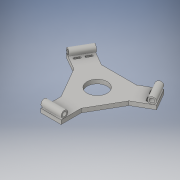
# Autodesk Inventor part: end effector
Saved by Autodesk Inventor 2016 (Build 200138000, 138)
## iProperties
Created: 2016-04-21
Part Number: end effector
Material: Generic
Document SubType Name: Modeling
Designer: Sam
Density: 1 g/cm^3
Appearance: Default
Author: Sam
Autodesk Inventor part; units mm, degrees
ref_plane "YZ Plane" through (0, 0, 0) normal (1, 0, 0) x (0, 1, 0)
ref_plane "XZ Plane" through (0, 0, 0) normal (0, 1, 0) x (-1, 0, 0)
ref_plane "XY Plane" through (0, 0, 0) normal (0, 0, 1) x (1, 0, 0)
sketch "Sketch1" plane through (0, 0, 0) normal (0, 1, 0) x (-1, 0, 0)
  line L0 (-7.5, 19.3301) -> (-7.5, 34.3301)
  line L1 (-7.5, 34.3301) -> (7.5, 34.3301)
  line L2 (7.5, 34.3301) -> (7.5, 19.3301)
  line L3 (20.4904, -3.1699) -> (33.4808, -10.6699)
  line L4 (33.4808, -10.6699) -> (25.9808, -23.6603)
  line L5 (25.9808, -23.6603) -> (12.9904, -16.1603)
  line L6 (-12.9904, -16.1603) -> (-25.9808, -23.6603)
  line L7 (-25.9808, -23.6603) -> (-33.4808, -10.6699)
  line L8 (-33.4808, -10.6699) -> (-20.4904, -3.1699)
  line L9 (7.5, 19.3301) -> (20.4904, -3.1699)
  line L10 (12.9904, -16.1603) -> (-12.9904, -16.1603)
  line L11 (-20.4904, -3.1699) -> (-7.5, 19.3301)
  point P0 (0, 0)
  point P1 (0, 0)
  constraints: 24 end point, 6 perpendicular, 1 coincident, 1 vertical, 1 other
extrude "Extrusion1" add sketch "Sketch1" along normal blind 3
sketch "Sketch2" plane through (0, 3, 0) normal (0, 1, 0) x (1, 0, 0)
  circle A0 centre (0, 0) radius 7.5
  line L0 (33.4808, 10.6699) -> (25.9808, 23.6603) projected
  line L1 (29.7308, 17.1651) -> (35.4808, 17.1651) construction
  line L2 (20.4904, 3.1699) -> (33.4808, 10.6699) projected
  line L3 (25.6261, 12.7745) -> (27.1261, 10.1764) construction
  line L4 (24.9766, 12.3995) -> (26.4766, 9.8014)
  line L5 (27.7756, 10.5514) -> (26.2756, 13.1495)
  arc A1 (26.2756, 13.1495) -> (24.9766, 12.3995) centre (25.6261, 12.7745) ccw
  arc A2 (26.4766, 9.8014) -> (27.7756, 10.5514) centre (27.1261, 10.1764) ccw
  line L6 (23.8761, 15.8056) -> (22.3761, 18.4037) construction
  line L7 (23.2266, 15.4306) -> (21.7266, 18.0287)
  line L8 (23.0256, 18.7787) -> (24.5256, 16.1806)
  arc A3 (23.2266, 15.4306) -> (24.5256, 16.1806) centre (23.8761, 15.8056) ccw
  arc A4 (23.0256, 18.7787) -> (21.7266, 18.0287) centre (22.3761, 18.4037) ccw
  line L9 (-23.2266, 15.4306) -> (-21.7266, 18.0287)
  arc A5 (-21.7266, 18.0287) -> (-23.0256, 18.7787) centre (-22.3761, 18.4037) ccw
  arc A6 (-24.5256, 16.1806) -> (-23.2266, 15.4306) centre (-23.8761, 15.8056) ccw
  line L10 (-23.8761, 15.8056) -> (-22.3761, 18.4037) construction
  line L11 (-23.0256, 18.7787) -> (-24.5256, 16.1806)
  arc A7 (-24.9766, 12.3995) -> (-26.2756, 13.1495) centre (-25.6261, 12.7745) ccw
  line L12 (-24.9766, 12.3995) -> (-26.4766, 9.8014)
  arc A8 (-27.7756, 10.5514) -> (-26.4766, 9.8014) centre (-27.1261, 10.1764) ccw
  line L13 (-27.7756, 10.5514) -> (-26.2756, 13.1495)
  line L14 (-29.7308, 17.1651) -> (-32.6058, 22.1447) construction
  line L15 (-25.6261, 12.7745) -> (-27.1261, 10.1764) construction
  line L16 (-1.75, -27.8301) -> (-4.75, -27.8301)
  arc A9 (-4.75, -27.8301) -> (-4.75, -29.3301) centre (-4.75, -28.5801) ccw
  arc A10 (-1.75, -29.3301) -> (-1.75, -27.8301) centre (-1.75, -28.5801) ccw
  line L17 (-1.75, -28.5801) -> (-4.75, -28.5801) construction
  line L18 (-4.75, -29.3301) -> (-1.75, -29.3301)
  arc A11 (1.75, -27.8301) -> (1.75, -29.3301) centre (1.75, -28.5801) ccw
  line L19 (1.75, -27.8301) -> (4.75, -27.8301)
  arc A12 (4.75, -29.3301) -> (4.75, -27.8301) centre (4.75, -28.5801) ccw
  line L20 (4.75, -29.3301) -> (1.75, -29.3301)
  line L21 (0, -34.3301) -> (-2.875, -39.3098) construction
  line L22 (1.75, -28.5801) -> (4.75, -28.5801) construction
  point P0 (26.3761, 11.4755)
  point P1 (23.1261, 17.1046)
  point P2 (-12.9904, 16.1603)
  point P3 (-23.1261, 17.1046)
  point P4 (-26.3761, 11.4755)
  point P5 (-25.9808, 23.6603)
  point P6 (-33.4808, 10.6699)
  point P7 (-7.5, -19.3301)
  point P8 (-3.25, -28.5801)
  point P9 (3.25, -28.5801)
  point P10 (-7.5, -34.3301)
  point P11 (7.5, -34.3301)
  dimension "d5" = 15
  dimension "d10" = 1.5
  dimension "d11" = 1.5
  dimension "d14" = 360
  constraints: 54 end point, 24 point on circle, 13 centre point, 4 tangent, 2 midpoint, 1 coincident, 1 horizontal, 1 parallel, 91 other
  measures "d5" diameter of A0
  measures "d10" distance of point (26.376, 11.475) L3.end
  measures "d11" diameter of A2
extrude "Extrusion2" cut sketch "Sketch2" against normal blind 3
sketch "Sketch3" plane through (0, 0, 0) normal (1, 0, 0) x (0, 1, 0)
  line L0 (3, 19.3301) -> (3, 34.3301) projected
  circle A0 centre (5.5, 31.8301) radius 2.5
  circle A1 centre (5.5, 31.8301) radius 1.55
  point P0 (0, 0)
  point P1 (3, 29.3301)
  dimension "d19" = 3.1
  constraints: 2 centre point, 1 coincident
  measures "d19" diameter of A1
extrude "Extrusion3" add sketch "Sketch3" along normal mid plane 15
pattern_circular "Circular Pattern1" count 3 over 360 about axis through (0, 3, 0) along (0, -1, 0) of "Extrusion3"
body "Solid1"
